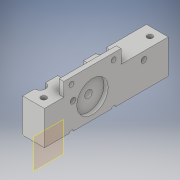
# Autodesk Inventor part: motorradrod
Saved by Autodesk Inventor 2019 (Build 230136000, 136)
## iProperties
Created: 2019-08-05
Part Number: motorradrod
Material: Generic
Document SubType Name: Modeling
Designer: rob
Density: 1 g/cm^3
Appearance: Default
Author: rob
Autodesk Inventor part; units mm, degrees
ref_plane "YZ Plane" through (0, 0, 0) normal (1, 0, 0) x (0, 1, 0)
ref_plane "XZ Plane" through (0, 0, 0) normal (0, 1, 0) x (-1, 0, 0)
ref_plane "XY Plane" through (0, 0, 0) normal (0, 0, 1) x (1, 0, 0)
sketch "Sketch1" plane through (0, 0, 0) normal (0, 1, 0) x (-1, 0, 0)
  line L0 (0, 0) -> (16, 0)
  line L1 (16, 0) -> (16, -91)
  line L2 (16, -91) -> (0, -91)
  line L3 (0, -91) -> (0, 0)
  dimension "d0" = 16
  dimension "d1" = 91
  constraints: 8 end point, 2 parallel, 1 horizontal, 1 perpendicular
  measures "d0" distance of L1.end L2.end
  measures "d1" distance of L0.end L1.end
extrude "Extrusion1" add sketch "Sketch1" along normal blind 25
sketch "Sketch2" plane through (0, 25, 0) normal (0, 1, 0) x (1, 0, 0)
  line L0 (-16, 91) -> (-16, 0) projected
  circle A0 centre (-16, 12.8045) radius 4
  circle A1 centre (-16, 57.8045) radius 4
  point P0 (0, 0)
  dimension "d4" = 8
  dimension "d5" = 8
  dimension "d6" = 45
  constraints: 2 centre point, 2 point on line
  measures "d4" diameter of A0
  measures "d5" diameter of A1
  measures "d6" distance of A1.centre A0.centre
extrude "Extrusion2" cut sketch "Sketch2" against normal blind 20
sketch "Sketch3" plane through (0, 25, 0) normal (0, 1, 0) x (1, 0, 0)
  circle A0 centre (-7, 6.5) radius 2
  circle A1 centre (-7, 84.5) radius 2
  line L0 (-16, 8.8045) -> (-16, 0) projected
  line L1 (-16, 53.8045) -> (-16, 16.8045) projected
  line L2 (-16, 8.8045) -> (-16, 61.8045) projected
  point P0 (0, 0)
  point P1 (-16, 3)
  point P2 (-16, 88)
  dimension "d10" = 4
  dimension "d12" = 4
  dimension "d15" = 9
  dimension "d17" = 9
  dimension "d18" = 6.5
  constraints: 2 centre point
  measures "d10" diameter of A0
  measures "d12" diameter of A1
  measures "d15" distance from line of L0 A0.centre
  measures "d17" distance from line of L2 A1.centre
  measures "d18" vertical distance of point (0, 0) A0.centre
ref_plane "Work Plane1" through (0, 0, -3) normal (1, 0, 0) x (0, 0, -1)
sketch "Sketch4" plane through (0, 0, -3) normal (1, 0, 0) x (0, 0, -1)
  circle A0 centre (17.9995, 19.5) radius 2
  circle A1 centre (69.9995, 19.5) radius 2
  line L0 (-3, 0) -> (88, 0) projected
  dimension "d21" = 4
  dimension "d22" = 4
  dimension "d34" = 52
  dimension "d59" = 19.5
  dimension "d60" = 19.5
  constraints: 2 centre point
  measures "d21" diameter of A0
  measures "d22" diameter of A1
  measures "d34" distance of A0.centre A1.centre
  measures "d59" distance from line of L0 A1.centre
  measures "d60" distance from line of L0 A0.centre
extrude "Extrusion4" cut sketch "Sketch4" against normal blind 30
sketch "Sketch5" plane through (-16, 0, -91) normal (-1, 0, 0) x (0, 0, 1)
  point P0 (91, 0)
sketch "Sketch6" plane through (-16, 0, -91) normal (-1, 0, 0) x (0, 0, 1)
  arc A0 (46.1955, 15) -> (65.1955, 15) centre (55.6955, 15) ccw
  line L0 (37.1955, 25) -> (37.1955, 5) projected
  line L1 (37.1955, 25) -> (74.1955, 25) projected
  line L2 (46.1955, 15) -> (46.1955, 30.0529)
  line L3 (46.1955, 30.0529) -> (65.1955, 30.0529)
  line L4 (65.1955, 30.0529) -> (65.1955, 15)
  point P0 (91, 0)
  dimension "d25" = 19
  dimension "d26" = 18.5
  dimension "d27" = 10
  constraints: 6 end point, 2 point on circle, 1 centre point, 1 parallel
  measures "d25" diameter of A0
  measures "d26" distance from line of L0 A0.centre
  measures "d27" distance from line of L1 A0.centre
extrude "Extrusion5" cut sketch "Sketch6" against normal blind 8.5
sketch "Sketch7" plane through (-7.5, 0, -91) normal (-1, 0, 0) x (0, 0, 1)
  circle A0 centre (55.6955, 15) radius 2.75
  line L0 (37.1955, 25) -> (37.1955, 5) projected
  point P0 (91, 0)
  dimension "d30" = 5.5
  dimension "d31" = 18.5
  constraints: 1 centre point
  measures "d30" diameter of A0
  measures "d31" distance from line of L0 A0.centre
extrude "Extrusion6" cut sketch "Sketch7" against normal blind 30
sketch "Sketch9" plane through (0, 25, 0) normal (0, 1, 0) x (1, 0, 0)
  line L0 (0, 14.304) -> (-3.5, 14.304)
  line L1 (-3.5, 14.304) -> (-3.5, 56.304)
  line L2 (-3.5, 56.304) -> (0, 56.304)
  line L3 (0, 56.304) -> (0, 14.304)
  line L4 (-16, 0) -> (0, 0) projected
  dimension "d48" = 3.5
  dimension "d49" = 42
  dimension "d50" = 14.304
  constraints: 8 end point, 2 parallel, 1 horizontal, 1 perpendicular
  measures "d48" distance of L1.end L2.end
  measures "d49" distance of L0.end L1.end
  measures "d50" distance between parallel lines of L4 L0
extrude "Extrusion7" add sketch "Sketch9" along normal blind 10
sketch "Sketch8" plane through (0, 0, 0) normal (1, 0, 0) x (0, 0, -1)
  circle A0 centre (19.8045, -0.5) radius 1.8
  circle A1 centre (50.8045, -0.5) radius 1.8
  circle A2 centre (50.8045, 30.5) radius 1.8
  circle A3 centre (19.8045, 30.5) radius 1.8
  circle A4 centre (35.3045, 15) radius 2.75 projected
  circle A5 centre (35.3045, 15) radius 11.5
  point P0 (0, 0)
  dimension "d35" = 3.6
  dimension "d36" = 3.6
  dimension "d37" = 3.6
  dimension "d38" = 3.6
  dimension "d39" = 31
  dimension "d40" = 31
  dimension "d41" = 31
  dimension "d42" = 31
  dimension "d43" = 0
  dimension "d44" = 23
  dimension "d45" = 15.5
  dimension "d46" = 15.5
  dimension "d47" = 0
  constraints: 5 centre point, 1 coincident
  measures "d35" diameter of A0
  measures "d36" diameter of A1
  measures "d37" diameter of A2
  measures "d38" diameter of A3
  measures "d39" distance of A2.centre A3.centre
  measures "d40" distance of A0.centre A3.centre
  measures "d41" distance of A1.centre A0.centre
  measures "d42" distance of A1.centre A2.centre
  measures "d43" vertical distance of A0.centre A1.centre
  measures "d44" diameter of A5
  measures "d45" horizontal distance of A3.centre A5.centre
  measures "d46" horizontal distance of A3.centre A5.centre
  measures "d47" horizontal distance of A3.centre A0.centre
extrude "Extrusion8" cut sketch "Sketch8" against normal blind 10 contours A0 | A1 | A2 | A3
extrude "Extrusion9" cut sketch "Sketch8" against normal blind 3 contours A5
extrude "Extrusion10" cut sketch "Sketch3" against normal blind 30
body "Solid1"
